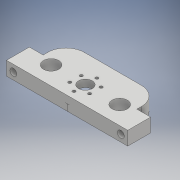
# Autodesk Inventor part: Base_Motor_acrilico_15
Saved by Autodesk Inventor 2017 (Build 210142000, 142)
## iProperties
Created: 2016-10-04
Part Number: Base_Motor_acrilico_15
Material: Generic
Document SubType Name: Modeling
Designer: ANDRES
Density: 1 g/cm^3
Appearance: Default
Author: ANDRES
Autodesk Inventor part; units mm, degrees
ref_plane "YZ Plane" through (0, 0, 0) normal (1, 0, 0) x (0, 1, 0)
ref_plane "XZ Plane" through (0, 0, 0) normal (0, 1, 0) x (-1, 0, 0)
ref_plane "XY Plane" through (0, 0, 0) normal (0, 0, 1) x (1, 0, 0)
sketch "Sketch1" plane through (0, 0, 0) normal (0, 0, 1) x (1, 0, 0)
  line L0 (-23.75, 0) -> (0, 0)
  circle A0 centre (0, 8) radius 8
  line L1 (0, 0) -> (23.75, 0)
  line L2 (12.5, 20) -> (-12.5, 20)
  circle A1 centre (15, 8) radius 3.35
  circle A2 centre (-15, 8) radius 3.35
  circle A3 centre (0, 8) radius 3
  line L3 (-23.75, 0) -> (-26.5, 0)
  line L4 (23.75, 0) -> (26.5, 0)
  line L5 (-26.5, 0) -> (-20.5, 0)
  line L6 (-20.5, 10) -> (-26.5, 10)
  line L7 (-26.5, 10) -> (-26.5, 0)
  line L8 (-20.5, 10) -> (-20.5, 12)
  line L9 (26.5, 0) -> (20.5, 0)
  line L10 (20.5, 10) -> (26.5, 10)
  line L11 (26.5, 10) -> (26.5, 0)
  line L12 (20.5, 10) -> (20.5, 12)
  arc A4 (-12.5, 20) -> (-20.5, 12) centre (-12.5, 12) ccw
  arc A5 (20.5, 12) -> (12.5, 20) centre (12.5, 12) ccw
  point P0 (20.5, 20)
  point P1 (-20.5, 20)
  dimension "d0" = 15
  dimension "d1" = 15
  dimension "d8" = 12
  dimension "d9" = 12
  dimension "d10" = 12
  dimension "d11" = 8
  dimension "d17" = 6.7
  dimension "d18" = 6.7
  dimension "d21" = 6
  dimension "d22" = 6
  dimension "d23" = 10
  dimension "d24" = 10
  dimension "d36" = 41
  dimension "d37" = 8
  dimension "d38" = 20
  dimension "d39" = 26.5
  dimension "d40" = 8
  constraints: 26 end point, 5 centre point, 5 point on line, 4 horizontal, 4 point on circle, 3 tangent, 2 parallel, 1 coincident, 1 vertical alignment, 1 other
  measures "d0" distance of point (0, 8) A2.centre
  measures "d1" distance of A1.centre point (0, 8)
  measures "d8" distance from line of L2 point (0, 8)
  measures "d9" distance from line of L2 A2.centre
  measures "d10" distance from line of L2 A1.centre
  measures "d11" distance from line of L1 A3.centre
  measures "d17" diameter of A2
  measures "d18" diameter of A1
  measures "d21" distance of L6.end L6.start
  measures "d22" distance of L10.start L10.end
  measures "d23" distance between parallel lines of L0 L6
  measures "d24" distance from line of L1.end L10
  measures "d36" distance between parallel lines of L12 L8
  measures "d37" radius of A4
  measures "d38" distance between parallel lines of L0 L2
  measures "d39" distance from line of L7 point (0, 0)
  measures "d40" radius of A5
ref_plane "Work Plane2" through (-26.5, 15, 0) normal (0, 1, 0) x (1, 0, 0)
sketch "Sketch2" plane through (-26.5, 15, 0) normal (0, 1, 0) x (1, 0, 0)
  line L0 (0, 0) -> (6, 0) projected
  line L1 (0, 0) -> (0, -6) projected
  line L2 (6, -6) -> (0, -6) projected
  line L3 (6, 0) -> (6, -6) projected
  line L4 (47, 0) -> (53, 0) projected
  line L5 (47, 0) -> (47, -6) projected
  line L6 (53, -6) -> (47, -6) projected
  line L7 (53, 0) -> (53, -6) projected
  circle A0 centre (3, -3) radius 1.5
  circle A1 centre (50, -3) radius 1.5
  point P0 (26.5, 0)
  dimension "d27" = 3
  dimension "d28" = 3
  constraints: 2 centre point
  measures "d27" diameter of A0
  measures "d28" diameter of A1
extrude "Extrusion3" add sketch "Sketch1" along normal blind 6 contours L3 L7 L6 L8 A4 L2 A5 L12 L10 L11 L4 L1 L0
hole "Hole2" at (-23.5, 15, 3) at (23.5, 15, 3) direction (0, -1, 0) diameter 3 end through all
sketch "Sketch3" plane through (0, 0, 6) normal (0, 0, 1) x (1, 0, 0)
  circle A0 centre (0, 8) radius 8 projected
  circle A1 centre (0, 13) radius 0.65
  circle A2 centre (-4.3301, 10.5) radius 0.65
  circle A3 centre (-4.3301, 5.5) radius 0.65
  circle A4 centre (0, 3) radius 0.65
  circle A5 centre (4.3301, 5.5) radius 0.65
  circle A6 centre (4.3301, 10.5) radius 0.65
  circle A7 centre (0, 8) radius 3
  point P0 (0, 0)
  dimension "d53" = 1.3
  dimension "d56" = 360
  dimension "d60" = 6
  constraints: 7 centre point, 2 coincident, 1 vertical alignment, 13 other
  measures "d53" diameter of A1
  measures "d60" diameter of A7
extrude "Extrusion6" add sketch "Sketch3" against normal blind 3.2
body "Solid3"
